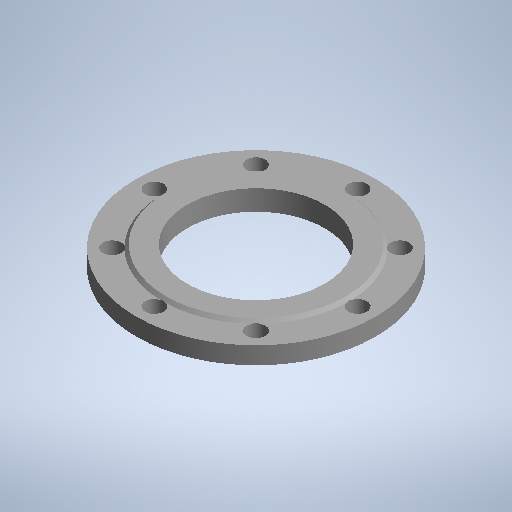
# Autodesk Inventor part: DMF Flange exit 2.0
Saved by Autodesk Inventor 2025 (Build 290162010, 162A)
## iProperties
Part Number: DMF Flange exit 2.0
Material: Generic
Document SubType Name: Sheet Metal
Designer: pokla
Appearance: Default
Sheet Metal Rule: Default_mm
Author: pokla
Autodesk Inventor part; units mm, degrees
ref_plane "YZ Plane" through (0, 0, 0) normal (1, 0, 0) x (0, 1, 0)
ref_plane "XZ Plane" through (0, 0, 0) normal (0, 1, 0) x (-1, 0, 0)
ref_plane "XY Plane" through (0, 0, 0) normal (0, 0, 1) x (1, 0, 0)
sketch "Sketch1" plane through (0, 0, 0) normal (0, 0, 1) x (1, 0, 0)
  line L0 (67.5, 20) -> (67.5, 0)
  line L1 (67.5, 0) -> (117.5, 0)
  line L2 (117.5, 0) -> (117.5, 17)
  line L3 (117.5, 17) -> (91.5, 17)
  line L4 (91.5, 17) -> (91.5, 20)
  line L5 (91.5, 20) -> (67.5, 20)
  line L6 (0, 0) -> (0, 46.5361)
  dimension "d0" = 50
  dimension "d1" = 24
  dimension "d2" = 135
  dimension "d3" = 17
  dimension "d4" = 20
  constraints: 14 end point, 5 perpendicular, 2 vertical, 1 horizontal alignment
  measures "d0" distance of L0.end L1.end
  measures "d1" distance of L4.end L0.start
  measures "d2" diameter of L0 L6
  measures "d3" distance of L1.end L2.end
  measures "d4" distance between parallel lines of L1 L5
revolve "Revolution1" add sketch "Sketch1" angle 360 about axis through (0, 0, 0) along (0, 1, 0)
chamfer "Chamfer1" distance 3 angle 45 1 edges at (-91.5, 20, 0)
sketch "Sketch2" plane through (0, 17, 0) normal (0, 1, 0) x (1, 0, 0)
  circle A0 centre (0, 0) radius 100
  point P0 (-100, 0)
  dimension "d9" = 200
  constraints: 2 horizontal alignment, 1 coincident, 2 other
hole "Hole1" at (-100, 17, 0) direction (0, -1, 0) diameter 18 end through all both
pattern_circular "Circular Pattern1" count 8 over 360 about axis through (0, 10, 0) along (0, 1, 0) of "Hole1"
body "Solid1"
